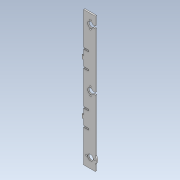
# Autodesk Inventor part: chassis_1_1_3
Saved by Autodesk Inventor 2022 (Build 260153000, 153)
## iProperties
Created: 2023-04-21
Part Number: chassis_1_1_3
Material: 一般
Document SubType Name: Modeling
Designer: JOU
Density: 1 g/cm^3
Appearance: 預設
Author: JOU
Autodesk Inventor part; units mm, degrees
ref_plane "YZ Plane" through (0, 0, 0) normal (1, 0, 0) x (0, 1, 0)
ref_plane "XZ Plane" through (0, 0, 0) normal (0, 1, 0) x (-1, 0, 0)
ref_plane "XY Plane" through (0, 0, 0) normal (0, 0, 1) x (1, 0, 0)
sketch "草圖1" plane through (0, 0, 0) normal (0, 0, 1) x (1, 0, 0)
  line L0 (-6, 142.5) -> (-10.5456, 142.5)
  arc A0 (-10.5456, 147.5) -> (-10.5456, 142.5) centre (-16, 145) ccw
  line L1 (-10.5456, 147.5) -> (-6, 147.5)
  circle A1 centre (-16, 153.5) radius 1.5
  circle A2 centre (-16, 136.5) radius 1.5
  circle A3 centre (-16, 275) radius 1.5
  circle A4 centre (-16, 258) radius 1.5
  circle A5 centre (-16, 23.5) radius 6
  circle A6 centre (-24.5, 23.5) radius 1.5
  circle A7 centre (-7.5, 23.5) radius 1.5
  line L2 (-6, 3) -> (-6, 16)
  line L3 (-6, 31) -> (-6, 142.5)
  arc A8 (-6, 16) -> (-6, 31) centre (-16, 23.5) ccw
  line L4 (-28.5, 3) -> (-28.5, 287)
  arc A9 (-10.546, 269.0008) -> (-10.546, 263.9992) centre (-16, 266.5) ccw
  line L5 (-28.5, 3) -> (-6, 3)
  line L6 (-6, 287) -> (-28.5, 287)
  line L7 (-6, 269.0008) -> (-10.546, 269.0008)
  line L8 (-10.546, 263.9992) -> (-6, 263.9992)
  line L9 (-6, 147.5) -> (-6, 263.9992)
  line L10 (-6, 269.0008) -> (-6, 287)
  circle A10 centre (-16, 23.5) radius 12.5 construction
  line L11 (-6, 72.05) -> (-6, 75)
  line L12 (-19.5, 74.2401) -> (-19.5, 72.05)
  line L13 (-19.5, 107.05) -> (-19.5, 110)
  line L14 (-6, 110) -> (-6, 107.05)
  line L15 (-6, 182.95) -> (-6, 180)
  line L16 (-6, 217.95) -> (-6, 215)
  line L17 (-19.5, 72.05) -> (-28.5, 72.05)
  line L18 (-28.5, 72.05) -> (-28.5, 75)
  line L19 (-28.5, 75) -> (-19.5, 75)
  line L20 (-19.5, 75) -> (-19.5, 72.05)
  line L21 (-19.5, 107.05) -> (-28.5, 107.05)
  line L22 (-28.5, 107.05) -> (-28.5, 110)
  line L23 (-28.5, 110) -> (-19.5, 110)
  line L24 (-19.5, 110) -> (-19.5, 107.05)
  line L25 (-19.5, 180) -> (-28.5, 180)
  line L26 (-28.5, 180) -> (-28.5, 182.95)
  line L27 (-28.5, 182.95) -> (-19.5, 182.95)
  line L28 (-19.5, 182.95) -> (-19.5, 180)
  line L29 (-28.5, 215) -> (-19.5, 215)
  line L30 (-19.5, 215) -> (-19.5, 217.95)
  line L31 (-19.5, 217.95) -> (-28.5, 217.95)
  line L32 (-28.5, 217.95) -> (-28.5, 215)
  point P0 (0, 0)
  point P1 (0, 0)
  dimension "d0" = 12
  dimension "d3" = 3
  dimension "d4" = 12
  dimension "d5" = 10
  dimension "d6" = 12.5
  dimension "d9" = 8.5
  dimension "d10" = 8.5
  dimension "d12" = 20.5
  dimension "d13" = 4.546
  dimension "d14" = 5.0015
  dimension "d27" = 70
  dimension "d28" = 35
  dimension "d29" = 35
  dimension "d30" = 70
  dimension "d31" = 2.95
  dimension "d32" = 9
  dimension "d33" = 2.95
  dimension "d34" = 2.95
  dimension "d35" = 2.95
  constraints: 66 end point, 11 parallel, 10 centre point, 9 horizontal, 8 point on line, 6 point on circle, 5 vertical, 4 collinear, 4 perpendicular, 2 coincident, 2 horizontal alignment, 1 equal radius, 22 other
  measures "d0" diameter of A5
  measures "d3" diameter of A6
  measures "d4" diameter of A9
  measures "d5" distance from line of L2 A8.centre
  measures "d6" radius of A8
  measures "d9" distance of A8.centre A6.centre
  measures "d10" distance of A8.centre A7.centre
  measures "d12" distance from line of A5.centre L5
  measures "d13" distance of L8.start L8.end
  measures "d14" distance between parallel lines of L8 L7
  measures "d27" distance from line of A0.centre L19
  measures "d28" distance from line of A0.centre L23
  measures "d29" distance from line of L25 A0.centre
  measures "d30" distance from line of A0.centre L29
  measures "d31" distance between parallel lines of L29 L31
  measures "d32" distance of L29.start L29.end
  measures "d33" distance between parallel lines of L25 L27
  measures "d34" distance between parallel lines of L19 L17
  measures "d35" distance between parallel lines of L23 L21
extrude "擠出1" add sketch "草圖1" along normal blind 3 contours L3 A8 L2 L5 L4 L17 L12 L20 L19 L21 L13 L23 L25 L28 L27 L29 L30 L31 L6 L10 L7 A9 L8 L9 L1 A0 L0
sketch "草圖2" plane through (0, 0, 0) normal (0, 0, -1) x (-1, 0, 0)
  line L0 (28.5, 287) -> (28.5, 217.95) projected
  line L1 (28.5, 287) -> (30.5, 287)
  line L2 (30.5, 287) -> (30.5, 217.95)
  line L3 (30.5, 217.95) -> (28.5, 217.95)
  line L4 (28.5, 217.95) -> (28.5, 287)
  line L5 (28.5, 215) -> (28.5, 182.95) projected
  line L6 (28.5, 215) -> (30.5, 215)
  line L7 (30.5, 215) -> (30.5, 182.95)
  line L8 (30.5, 182.95) -> (28.5, 182.95)
  line L9 (28.5, 182.95) -> (28.5, 215)
  line L10 (28.5, 180) -> (28.5, 110) projected
  line L11 (28.5, 180) -> (30.5, 180)
  line L12 (30.5, 180) -> (30.5, 110)
  line L13 (30.5, 110) -> (28.5, 110)
  line L14 (28.5, 110) -> (28.5, 180)
  line L15 (28.5, 107.05) -> (28.5, 75) projected
  line L16 (28.5, 107.05) -> (30.5, 107.05)
  line L17 (30.5, 107.05) -> (30.5, 75)
  line L18 (30.5, 75) -> (28.5, 75)
  line L19 (28.5, 75) -> (28.5, 107.05)
  line L20 (19.5, 72.05) -> (28.5, 72.05) projected
  line L21 (28.5, 72.05) -> (30.5, 72.05)
  line L22 (30.5, 72.05) -> (30.5, 3)
  line L23 (30.5, 3) -> (28.5, 3)
  line L24 (28.5, 3) -> (28.5, 72.05)
  line L25 (28.5, 182.95) -> (19.5, 182.95) projected
  line L26 (28.5, 110) -> (19.5, 110) projected
  line L27 (28.5, 75) -> (19.5, 75) projected
  line L28 (28.5, 3) -> (6, 3) projected
  point P0 (0, 0)
  dimension "d36" = 2
  constraints: 40 end point, 10 parallel, 6 collinear, 5 horizontal, 5 perpendicular, 2 point on line
  measures "d36" distance between parallel lines of L24 L22
extrude "擠出2" add sketch "草圖2" against normal up to surface (3 mm away)
sketch "草圖3" plane through (0, 0, 0) normal (0, 0, -1) x (-1, 0, 0)
  line L0 (33.5, 203) -> (30.5, 203)
  line L1 (30.5, 203) -> (30.5, 195)
  line L2 (30.5, 195) -> (33.5, 195)
  line L3 (33.5, 195) -> (33.5, 203)
  line L4 (33.5, 95) -> (30.5, 95)
  line L5 (30.5, 95) -> (30.5, 87)
  line L6 (30.5, 87) -> (33.5, 87)
  line L7 (33.5, 87) -> (33.5, 95)
  line L8 (30.5, 75) -> (30.5, 107.05) projected
  line L9 (30.5, 182.95) -> (30.5, 215) projected
  line L10 (19.5, 215) -> (30.5, 215) projected
  point P0 (0, 0)
  dimension "d39" = 8
  dimension "d40" = 8
  dimension "d41" = 3
  dimension "d42" = 3
  dimension "d43" = 12
  dimension "d44" = 100
  constraints: 16 end point, 4 parallel, 2 collinear, 2 horizontal, 2 perpendicular
  measures "d39" distance of L6.end L4.start
  measures "d40" distance between parallel lines of L0 L2
  measures "d41" distance between parallel lines of L5 L7
  measures "d42" distance between parallel lines of L1 L3
  measures "d43" distance between parallel lines of L10 L0
  measures "d44" distance between parallel lines of L4 L2
extrude "擠出3" add sketch "草圖3" against normal up to surface (3 mm away)
